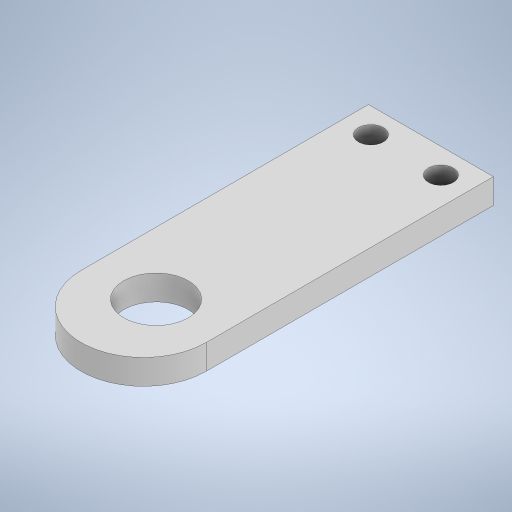
# Autodesk Inventor part: self aligning bearing holder
Saved by Autodesk Inventor 2023 (Build 270158000, 158)
## iProperties
Created: 2023-01-25
Part Number: self aligning bearing holder
Material: Generic
Document SubType Name: Modeling
Designer: rosam
Density: 1 g/cm^3
Appearance: Default
Author: rosam
Autodesk Inventor part; units mm, degrees
ref_plane "YZ Plane" through (0, 0, 0) normal (1, 0, 0) x (0, 1, 0)
ref_plane "XZ Plane" through (0, 0, 0) normal (0, 1, 0) x (-1, 0, 0)
ref_plane "XY Plane" through (0, 0, 0) normal (0, 0, 1) x (1, 0, 0)
sketch "Sketch1" plane through (0, 0, 0) normal (0, 1, 0) x (-1, 0, 0)
  line L0 (22.1143, 19.9744) -> (22.1143, -53.0506)
  line L1 (22.1143, -53.0506) -> (-9.6357, -53.0506)
  line L2 (-9.6357, -53.0506) -> (-9.6357, 19.9744)
  arc A0 (22.1143, 19.9744) -> (-9.6357, 19.9744) centre (6.2393, 19.9744) ccw
  circle A1 centre (15.1293, -46.7006) radius 3.175
  circle A2 centre (-2.6507, -46.7006) radius 3.175
  circle A3 centre (6.2393, 16.7994) radius 8.1915
  point P0 (0, 0)
  point P1 (6.2393, 35.8494)
  dimension "d0" = 31.75
  dimension "d1" = 88.9
  dimension "d3" = 6.35
  dimension "d4" = 6.35
  dimension "d5" = 17.78
  dimension "d6" = 6.35
  dimension "d7" = 6.35
  dimension "d10" = 6.985
  dimension "d11" = 6.985
  dimension "d12" = 16.383
  dimension "d14" = 3.175
  dimension "d15" = 15.875
  dimension "d16" = 15.875
  constraints: 6 end point, 4 centre point, 3 point on circle, 2 perpendicular, 2 tangent, 1 vertical
  measures "d0" distance of L0.end L1.end
  measures "d1" distance from line of L1 point (6.239, 35.849)
  measures "d3" diameter of A1
  measures "d4" diameter of A2
  measures "d5" distance of A1.centre A2.centre
  measures "d6" distance from line of L1 A1.centre
  measures "d7" distance from line of L1 A2.centre
  measures "d10" distance from line of L2 A2.centre
  measures "d11" distance from line of L0 A1.centre
  measures "d12" diameter of A3
  measures "d14" distance of A0.centre A3.centre
  measures "d15" distance from line of L0 A3.centre
  measures "d16" distance from line of L2 A3.centre
extrude "Extrusion2" add sketch "Sketch1" along normal blind 6.35
equation "\"d7\" = d6"
equation "\"d10\" = d11"
equation "\"d15\" = d16"
body "Solid2"
